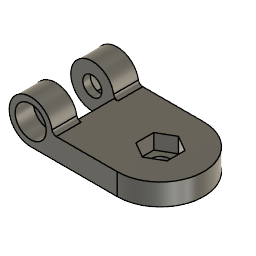
Hinge (Autodesk Fusion 360 archive; units mm, degrees)
design "Hinge Top"
part number: 2026-01-11-23-29-48-770
Autodesk Fusion 360 part; units mm, degrees
sketch "Sketch1" plane through (0, 0, 0) normal (0, 1, 0) x (1, 0, 0)
  line L0 (-20, 0) -> (20, 0)
  line L1 (20, 0) -> (20, -5)
  line L2 (20, -5) -> (-20, -5)
  line L3 (-20, -5) -> (-20, 0)
  circle A0 centre (0, -5) radius 5
  circle A1 centre (0, -5) radius 3.6
  circle A2 centre (0, -5) radius 2.2
  dimension "d19" = 10
  dimension "d20" = 7.2
  dimension "d21" = 4.4
  constraint horizontal L0
  constraint vertical L1
  constraint horizontal L2
  constraint vertical L3
  constraint midpoint L2 A0.centre
  constraint concentric A0 A1
  constraint concentric A1 A2
  measures "d19" diameter of A0
  measures "d20" diameter of A1
  measures "d21" diameter of A2
extrude "Extrude6" add sketch "Sketch1" along normal blind 5 contours L0 L1 L2 A0 | L2 A0 A1 | L2 A0 A1 | L2 A1 A2 | L2 A1 A2
sketch "Sketch2" plane through (0, 0, 0) normal (0, -1, 0) x (1, 0, 0)
  circle A0 centre (0, 5) radius 2.2
  arc A1 (5, 5) -> (0, 0) centre (0, 5) ccw
  line L0 (0, 0) -> (20, 0)
  line L1 (20, 0) -> (20, 5)
  line L2 (20, 5) -> (5, 5)
  circle A2 centre (0, 5) radius 3.6
  dimension "d24" = 7.2
  constraint concentric A0 A2
  measures "d24" diameter of A2
extrude "Extrude7" cut sketch "Sketch2" against normal blind 4.2 contours A2
sketch "Sketch3" plane through (0, 5, 0) normal (0, 1, 0) x (-1, 0, 0)
  circle A0 centre (0, 5) radius 2.2
  arc A1 (0, 0) -> (-5, 5) centre (0, 5) ccw
  line L0 (-5, 5) -> (-20, 5)
  line L1 (-20, 5) -> (-20, 0)
  line L2 (-20, 0) -> (0, 0)
  circle A2 centre (0, 5) radius 5
  constraint concentric A0 A2
  constraint coincident A1.end A2
extrude "Extrude8" add sketch "Sketch3" along normal blind 10 contours L0 L1 L2 A2
sketch "Sketch4" plane through (0, 15, 0) normal (0, 1, 0) x (-1, 0, 0)
  line L0 (-5, 5) -> (-20, 5)
  line L1 (-20, 5) -> (-20, 0)
  line L2 (-20, 0) -> (0, 0)
  arc A0 (-5, 5) -> (0, 0) centre (0, 5) ccw
  circle A1 centre (0, 5) radius 5
  line L3 (-2.0785, 8.6) -> (-4.1569, 5)
  line L4 (-4.1569, 5) -> (-2.0785, 1.4)
  line L5 (-2.0785, 1.4) -> (2.0785, 1.4)
  line L6 (2.0785, 1.4) -> (4.1569, 5)
  line L7 (4.1569, 5) -> (2.0785, 8.6)
  line L8 (2.0785, 8.6) -> (-2.0785, 8.6)
  circle A2 centre (0, 5) radius 2.2
  point P0 (0, 5)
  dimension "d34" = 3.6
  dimension "d35" = 4.4
  constraint concentric A0 A1
  constraint coincident L0.start A1
  constraint coincident P0 A0.centre
  constraint concentric A1 A2
  measures "d34" distance of P0 L8
  measures "d35" diameter of A2
extrude "Extrude11" add sketch "Sketch4" along normal blind 5 contours L0 L1 L2 A0 A1 | A0 A1
extrude "Extrude12" add sketch "Sketch4" along normal blind 1 contours L3 L4 L5 L6 L7 L8
fillet "Fillet4" radius 1 2 edges at (5, 17.5, 5) (5, 2.5, 5)
sketch "Sketch9" plane through (0, 0, 5) normal (0, 0, 1) x (-1, 0, 0)
  line L0 (-20, 0) -> (-20, -20)
  line L1 (-20, -20) -> (-5.9161, -20)
  line L2 (-5.9161, -20) -> (-5.9161, -15)
  line L3 (-5.9161, -15) -> (-5, -15)
  line L4 (-5, -15) -> (-5, -5)
  line L5 (-5, -5) -> (-5.9161, -5)
  line L6 (-5.9161, -5) -> (-5.9161, 0)
  line L7 (-5.9161, 0) -> (-20, 0)
  circle A0 centre (-20, -10) radius 10
  line L8 (-16.4, -7.9215) -> (-20, -5.8431)
  line L9 (-20, -5.8431) -> (-23.6, -7.9215)
  line L10 (-23.6, -7.9215) -> (-23.6, -12.0785)
  line L11 (-23.6, -12.0785) -> (-20, -14.1569)
  line L12 (-20, -14.1569) -> (-16.4, -12.0785)
  line L13 (-16.4, -12.0785) -> (-16.4, -7.9215)
  circle A1 centre (-20, -10) radius 2.2
  point P0 (-20, -10)
  dimension "d100" = 20
  dimension "d103" = 3.6
  dimension "d104" = 4.4
  constraint midpoint L0 P0
  constraint coincident P0 A0.centre
  constraint concentric A0 A1
  measures "d100" diameter of A0
  measures "d103" distance of P0 L13
  measures "d104" diameter of A1
move_body "Move2" bodies 1 to x (1, 0, 0) y (0, 1, 0) z (0, 0, 1) at (15, 0, 0)
move_body "Move3" bodies 1 to x (1, 0, 0) y (0, 1, 0) z (0, 0, 1) at (-15, 0, 0)
extrude "Extrude21" add 1 faces at (-0.2983, 15, 0.9533) along direction (0, -1, 0) blind 0.8
extrude "Extrude22" add 1 faces at (-0.2983, 5, 0.9533) along direction (0, 1, 0) blind 0.8
extrude "Extrude23" add 1 faces at (-0.2983, 14.2, 0.9533) along direction (0, -1, 0) blind 0.1
extrude "Extrude24" add 1 faces at (-0.2983, 5.8, 0.9533) along direction (0, 1, 0) blind 0.1
extrude "Extrude26" cut 1 faces at (-0.2983, 5.9, 0.9533) along direction (0, -1, 0) blind 0.15
extrude "Extrude27" cut 1 faces at (-0.2983, 14.1, 0.9533) along direction (0, 1, 0) blind 0.15
extrude "Extrude28" add sketch "Sketch9" against normal blind 5 contours L0 A0 L9 L10 L11 | L0 L9 L10 L11 A1 | L0 A1 picked at (-20.3255, -9.2911)
extrude "Extrude29" cut sketch "Sketch9" against normal blind 3.5 contours L0 L8 L12 L13 A1 | L0 L9 L10 L11 A1
extrude "Extrude30" cut sketch "Sketch9" against normal through all contours L0 A1 | L0 A1

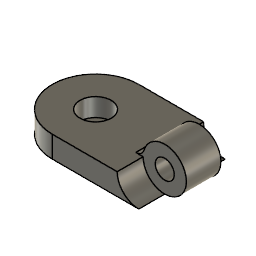
design "Hinge Bottom"
part number: 2026-01-11-23-29-48-770
Autodesk Fusion 360 part; units mm, degrees
sketch "Sketch1" plane through (0, 0, 0) normal (0, 1, 0) x (1, 0, 0)
  line L0 (-20, 0) -> (20, 0)
  line L1 (20, 0) -> (20, -5)
  line L2 (20, -5) -> (-20, -5)
  line L3 (-20, -5) -> (-20, 0)
  circle A0 centre (0, -5) radius 5
  circle A1 centre (0, -5) radius 3.6
  circle A2 centre (0, -5) radius 2.2
  dimension "d19" = 10
  dimension "d20" = 7.2
  dimension "d21" = 4.4
  constraint horizontal L0
  constraint vertical L1
  constraint horizontal L2
  constraint vertical L3
  constraint midpoint L2 A0.centre
  constraint concentric A0 A1
  constraint concentric A1 A2
  measures "d19" diameter of A0
  measures "d20" diameter of A1
  measures "d21" diameter of A2
extrude "Extrude13" add sketch "Sketch1" along normal blind 20 contours L0 L2 L3 A0
extrude "Extrude14" add sketch "Sketch1" along normal blind 15 contours L2 A0 A1 | L2 A0 A1 | L2 A1 A2 | L2 A1 A2
sketch "Sketch8" plane through (0, 0, 0) normal (0, -1, 0) x (1, 0, 0)
  circle A0 centre (0, 5) radius 2.2
  line L0 (-20, 0) -> (0, 0)
  arc A1 (0, 0) -> (-5, 5) centre (0, 5) ccw
  line L1 (-5, 5) -> (-20, 5)
  circle A2 centre (0, 5) radius 5
  line L2 (-20, 5) -> (-20, 0)
  constraint concentric A0 A2
  constraint coincident A1.end A2
extrude "Extrude15" cut sketch "Sketch8" against normal blind 5 contours A1 A2
extrude "Extrude21" cut 1 faces at (0.2994, 15, 0.9534) along direction (0, -1, 0) blind 1
extrude "Extrude22" cut 1 faces at (0.2994, 5, 0.9534) along direction (0, 1, 0) blind 1
sketch "Sketch12" plane through (0, 0, 5) normal (0, 0, 1) x (-1, 0, 0)
  line L0 (20, 0) -> (5, 0)
  line L1 (5, 0) -> (5, -6)
  line L2 (5, -6) -> (5, -14)
  line L3 (5, -14) -> (5, -20)
  line L4 (5, -20) -> (20, -20)
  line L5 (20, -20) -> (20, 0)
  circle A0 centre (20, -10) radius 10
  circle A1 centre (20, -10) radius 3.6
  circle A2 centre (20, -10) radius 2.2
  dimension "d92" = 20
  dimension "d95" = 7.2
  dimension "d96" = 4.4
  constraint midpoint L5 A0.centre
  constraint concentric A0 A1
  constraint concentric A1 A2
  measures "d92" diameter of A0
  measures "d95" diameter of A1
  measures "d96" diameter of A2
extrude "Extrude24" add sketch "Sketch12" against normal blind 5 contours L5 A0 A1 | L5 A1 A2 | L5 A2 picked at (27.8205, -10.6452) picked at (23.1211, -10.1708) picked at (20.6671, -9.6954)
extrude "Extrude25" cut sketch "Sketch12" against normal blind 4.2 contours L5 A1 A2 | L5 A1 A2
extrude "Extrude26" cut sketch "Sketch12" against normal through all contours L5 A2 | L5 A2
fillet "Fillet13" radius 2 1 edges at (-5, 10, 5)

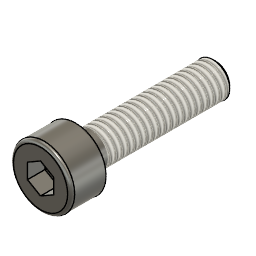
design "Hexagon Socket Head Cap Screw ISO 4762 - M4 x 16 Steel 4.6 Plain"
description: Hexagon Socket Head Cap Screw ISO 4762 - M4 x 16
part number: ISO 4762 - M4 x 16 Steel 4.6 Plain
Autodesk Fusion 360 part; units mm, degrees
sketch "Sketch1" plane through (0, 0, 0) normal (0, 1, 0) x (1, 0, 0)
  line L0 (-2, 0) -> (-2, 16)
  line L1 (-2, 16) -> (0, 16)
  line L2 (0, 16) -> (0, -4)
  line L3 (-2, 0) -> (-3.5, 0)
  line L4 (-3.5, 0) -> (-3.5, -4)
  line L5 (-3.5, -4) -> (0, -4)
  dimension "d9" = 4
  dimension "d106" = 4
  dimension "d107" = 16
  dimension "d116" = 7
  constraint perpendicular L0 L1
  constraint collinear origin L1.end L2.end
  constraint perpendicular L0 L3
  constraint coincident origin L3
  constraint vertical L2
  constraint coincident L2 L5.end
  constraint perpendicular L2 L5
  measures "d106" distance of L3 L5
  measures "d107" distance of origin L1
revolve "Revolve1" add sketch "Sketch1" angle 360 about axis through (0, 0, -16) along (0, 0, 1)
ref_plane "WorkPlane1" through (0, 0, 4) normal (0, 0, 1) x (1, 0, 0)
sketch "Sketch6" plane through (0, 0, 4) normal (0, 0, 1) x (1, 0, 0)
  line L0 (-1.5, 0.866) -> (-1.5, -0.866)
  line L1 (-1.5, -0.866) -> (0, -1.7321)
  line L2 (0, -1.7321) -> (1.5, -0.866)
  line L3 (1.5, -0.866) -> (1.5, 0.866)
  line L4 (1.5, 0.866) -> (0, 1.7321)
  line L5 (0, 1.7321) -> (-1.5, 0.866)
  dimension "d117" = 3
  constraint vertical L0
  measures "d117" distance of L0 L3
extrude "Extrude1" cut sketch "Sketch6" against normal blind 2
extrude "Extrude2" cut 1 faces at (-0.5, 0.2887, 2) along direction (0, 0, -1) blind 2 draft -85
fillet "Fillet4" radius 0.4 1 edges at (-3.2631, 1.2657, 4)
thread "Thread3" "ISO Metric profile 4.0 M4x0.7 M4x0.7 6g" major diameter 3.908 minor diameter 3.111 pitch 0.7 angle 60 resizes the face on face at (-1.9901, 0.1991, -10.6667) from (0, 0, -1.75) to (0, 0, -16)
sketch "Sketch7" plane through (0, 0, 0) normal (0, 1, 0) x (1, 0, 0)
  line L0 (-2.04, 16) -> (-2.04, 15.6)
  line L1 (-2.04, 15.6) -> (-1.64, 16)
  line L2 (0, 16) -> (0, -4)
  line L3 (-2.04, 16) -> (0, 16)
  dimension "d101" = 45
  dimension "d112" = 0.4
  dimension "d113" = 2.04
  constraint coincident L2.start L3.end
  constraint perpendicular L2 L3
  constraint coincident L1.end L3
  constraint perpendicular L0 L3
  measures "d101" angle of L0 L1
  measures "d112" distance of L0.end L3
  measures "d113" distance of L0 L2.start
revolve "Revolve3" cut sketch "Sketch7" angle 360 about axis through (0, 0, 1.75) along (0, 0, 1)
equation "d9 = adsk_nomdia"
equation "adsk_nomlen = 16.00 mm"
equation "adsk_headh = 4.00 mm"
equation "adsk_headdia = 7.00 mm"
equation "adsk_nomdia = 4.00 mm"
equation "adsk_philwidth = 3.00 mm"
equation "d31 = -adsk_phildepth"
equation "adsk_phildepth = 2.00 mm"
equation "d71 = adsk_headh"
equation "d76 = -adsk_phildepth"
equation "adsk_thrlen = 14.25 mm"
equation "d86 = adsk_nomdia * 0.1"
equation "adsk_startang = 45.00 deg"
equation "d101 = adsk_startang"
equation "adsk_pitch1 = 0.70 mm"
equation "adsk_startlen = 0.40 mm"
equation "d106 = adsk_headh"
equation "d107 = adsk_nomlen"
equation "d112 = adsk_startlen"
equation "d113 = adsk_nomdia * 0.51"
equation "d115 = min(adsk_thrlen; adsk_nomlen - 0.001 mm)"
equation "d116 = adsk_headdia"
equation "d117 = adsk_philwidth"

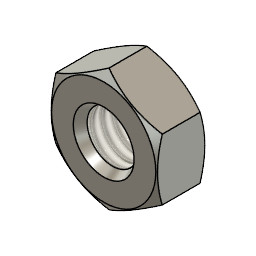
design "Hexagon Regular Nut ISO 4032 - M4 Steel 6 Plain"
description: Hexagon Regular Nut ISO 4032 - M4
part number: ISO 4032 - M4 Steel 6 Plain
Autodesk Fusion 360 part; units mm, degrees
sketch "Sketch1" plane through (0, 0, 0) normal (0, 1, 0) x (1, 0, 0)
  line L0 (0, 0) -> (0, -3.2)
  line L1 (-2, 0) -> (-3.43, 0)
  line L2 (-3.43, 0) -> (-4.0425, -0.3536)
  line L3 (-4.0425, -0.3536) -> (-4.0425, -2.8464)
  line L4 (-4.0425, -2.8464) -> (-3.43, -3.2)
  line L5 (-3.43, -3.2) -> (-2, -3.2)
  line L6 (-2, -3.2) -> (-2, 0)
  dimension "d121" = 4
  dimension "d122" = 30
  dimension "d123" = 30
  dimension "d128" = 8.085
  dimension "d172" = 6.86
  dimension "d179" = 3.2
  constraint vertical L0
  constraint coincident L0 L0.end
  constraint coincident origin L0
  constraint horizontal L1
  constraint coincident L0.start L1
  constraint coincident L0.start origin
  constraint coincident L0.end L5
  constraint vertical L1.end L4.end
  measures "d122" angle of L1 L2
  measures "d123" angle of L4 L5
  measures "d179" distance of L1 L5
revolve "Revolve1" add sketch "Sketch1" angle 360 about axis through (0, 0, 0) along (0, 0, 1)
sketch "Sketch8" plane through (0, 0, 3.2) normal (0, 0, 1) x (1, 0, 0)
  line L0 (-3.5, -2.0228) -> (-3.5, 2.0228)
  circle A0 centre (0, 0) radius 2
  circle A1 centre (0, 0) radius 4.0425
  dimension "d114" = 3.5
  constraint coincident L0.end A1
  constraint coincident L0.start A1
  constraint vertical L0
  measures "d114" distance of A0.centre L0
extrude "Extrude5" cut sketch "Sketch8" against normal blind 3.2 contours L0 A1 picked at (-3.5875, 0.4927)
pattern_circular "C-Pattern2" count 6 over 360 about axis through (0, 0, 1.75) along (0, 0, 1) of "Extrude5"
thread "Thread3" "ISO Metric profile 4.0 M4x0.7 M4x0.7 6H" major diameter 4.1095 minor diameter 3.332 pitch 0.7 angle 60 resizes the face on face at (-1.9975, 0.0997, 2.1333)
sketch "Sketch12" plane through (0, 0, 0) normal (0, 1, 0) x (1, 0, 0)
  line L0 (-2, 0) -> (0, 0)
  line L1 (-1.0762, -1.6) -> (-2, 0)
  line L2 (-2, -3.2) -> (0, -3.2)
  line L3 (-1.0762, -1.6) -> (-2, -3.2)
  line L4 (0, 0) -> (0, -3.2)
  dimension "d169" = 60
  dimension "d177" = 2
  dimension "d178" = 60
  constraint horizontal L0
  constraint coincident L1.start L3.start
  constraint vertical L0.start L2.start
  constraint coincident L2.end L4.end
  constraint coincident L0.end L4.start
  constraint perpendicular L2 L4
  measures "d169" angle of L2 L3
  measures "d177" distance of L0.start L4
  measures "d178" angle of L0 L1
revolve "Revolve3" cut sketch "Sketch12" angle 360 about axis through (0, 0, 1.75) along (0, 0, 1)
equation "adsk_nheig = 3.20 mm"
equation "adsk_maxdia = 8.085 mm"
equation "adsk_nomdia = 4.00 mm"
equation "d89 = -adsk_nheig"
equation "adsk_waflat = 7.00 mm"
equation "d114 = adsk_waflat / 2"
equation "adsk_chamang1 = 30.00 deg"
equation "adsk_chamang2 = 30.00 deg"
equation "d121 = adsk_nomdia"
equation "d122 = adsk_chamang1"
equation "d123 = adsk_chamang2"
equation "d128 = adsk_maxdia"
equation "d163 = adsk_nheig"
equation "adsk_beardia = 6.86 mm"
equation "d172 = adsk_beardia"
equation "d177 = adsk_nomdia * 0.5"
equation "d179 = adsk_nheig"
